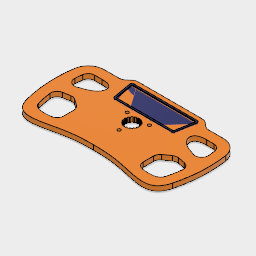
FSAE Steering Wheel 4_CSA011020 (Autodesk Fusion 360 design; units mm, degrees)
Autodesk Fusion 360 part; units mm, degrees
note: some values were not read from the file. Set by a fixed rule: which sketch regions a step uses.
sketch "Main Plate" plane through (0, 0, 0) normal (0, 1, 0) x (1, 0, 0) in component "Steering Wheel Base Plate"
  line L0 (-152.4, 0) -> (152.4, 0) construction
  line L1 (0, -76.2) -> (0, 76.2) construction
  line L2 (0, 76.2) -> (63.5, 76.2)
  line L3 (0, -76.2) -> (-8.4964, -76.2) construction
  arc A0 (144.3344, -63.5) -> (144.3344, 63.5) centre (-101.6, 0) ccw
  line L4 (88.9, 63.5) -> (144.3344, 63.5)
  spline S0 degree 5 poles (63.5, 76.2) (64.7871, 76.2) (67.2229, 75.9407) (70.4619, 74.7744) (74.1142, 71.971) (78.2858, 67.729) (81.9381, 64.9256) (85.1771, 63.7593) (87.6129, 63.5) (88.9, 63.5) knots 0 0 0 0 0 0 0.2 0.4 0.6 0.8 1 1 1 1 1 1
  spline S1 degree 5 poles (0, -76.2) (4.2797, -76.2) (12.5023, -76.2824) (23.8251, -76.6531) (37.1715, -77.6792) (52.2799, -79.9533) (67.2956, -83.1876) (83.1544, -86.9749) (99.9496, -90.4235) (115.5574, -91.6209) (128.6696, -88.7753) (136.6498, -82.0535) (141.0961, -74.0037) (143.3701, -67.235) (144.3344, -63.5) knots 0 0 0 0 0 0 0.1 0.2 0.3 0.4 0.5 0.6 0.7 0.8 0.9 1 1 1 1 1 1
  line L5 (139.5719, -81.9451) -> (149.097, -45.0549)
  line L6 (103.5148, 10.8591) -> (133.35, 0)
  arc A1 (133.35, 0) -> (129.107, 44.45) centre (-101.6, 0) ccw
  line L7 (103.707, 44.45) -> (129.107, 44.45)
  spline S2 degree 5 poles (103.707, 44.45) (99.6383, 44.45) (92.5553, 43.9266) (85.0911, 41.5729) (80.6953, 35.8381) (82.1279, 26.5542) (87.7958, 19.214) (94.5954, 14.5846) (100.3396, 12.0148) (103.5148, 10.8591) knots 0 0 0 0 0 0 0.2 0.4 0.6 0.8 1 1 1 1 1 1
  line L8 (113.232, 44.45) -> (94.182, 44.45)
  line L9 (-19.05, -76.2) -> (19.05, -76.2)
  line L10 (77.9006, -86.1433) -> (109.1683, -91.6567)
  line L11 (78.9249, -29.21) -> (78.9249, -67.31)
  arc A2 (125.8894, -58.7375) -> (132.5764, -19.05) centre (-101.6, 0) ccw
  line L12 (132.5764, -19.05) -> (101.3088, -13.5367)
  line L13 (101.3088, -13.5367) -> (78.9249, -29.21)
  spline S3 degree 5 poles (125.8894, -58.7375) (125.4726, -60.3516) (124.3156, -63.2508) (121.6104, -66.613) (116.2467, -69.3606) (106.9918, -70.6255) (97.452, -70.2137) (88.8277, -69.0979) (82.3477, -67.97) (78.9249, -67.31) knots 0 0 0 0 0 0 0.2 0.4 0.6 0.8 1 1 1 1 1 1
  line L14 (86.5574, -68.7817) -> (71.2925, -65.8383)
  line L15 (126.6342, -55.8526) -> (125.1445, -61.6224)
  line L16 (0, 76.2) -> (-63.5, 76.2)
  spline S4 degree 5 poles (-63.5, 76.2) (-64.7871, 76.2) (-67.2229, 75.9407) (-70.4619, 74.7744) (-74.1142, 71.971) (-78.2858, 67.729) (-81.9381, 64.9256) (-85.1771, 63.7593) (-87.6129, 63.5) (-88.9, 63.5) knots 0 0 0 0 0 0 0.2 0.4 0.6 0.8 1 1 1 1 1 1
  line L17 (-88.9, 63.5) -> (-144.3344, 63.5)
  spline S5 degree 5 poles (-103.707, 44.45) (-99.6383, 44.45) (-92.5553, 43.9266) (-85.0911, 41.5729) (-80.6953, 35.8381) (-82.1279, 26.5542) (-87.7958, 19.214) (-94.5954, 14.5846) (-100.3396, 12.0148) (-103.5148, 10.8591) knots 0 0 0 0 0 0 0.2 0.4 0.6 0.8 1 1 1 1 1 1
  line L18 (-113.232, 44.45) -> (-94.182, 44.45)
  line L19 (-103.707, 44.45) -> (-129.107, 44.45)
  arc A3 (-129.107, 44.45) -> (-133.35, 0) centre (101.6, 0) ccw
  line L20 (-103.5148, 10.8591) -> (-133.35, 0)
  arc A4 (-144.3344, 63.5) -> (-144.3344, -63.5) centre (101.6, 0) ccw
  spline S6 degree 5 poles (0, -76.2) (-4.2797, -76.2) (-12.5023, -76.2824) (-23.8251, -76.6531) (-37.1715, -77.6792) (-52.2799, -79.9533) (-67.2956, -83.1876) (-83.1544, -86.9749) (-99.9496, -90.4235) (-115.5574, -91.6209) (-128.6696, -88.7753) (-136.6498, -82.0535) (-141.0961, -74.0037) (-143.3701, -67.235) (-144.3344, -63.5) knots 0 0 0 0 0 0 0.1 0.2 0.3 0.4 0.5 0.6 0.7 0.8 0.9 1 1 1 1 1 1
  line L21 (19.05, -76.2) -> (-19.05, -76.2)
  line L22 (-77.9006, -86.1433) -> (-109.1683, -91.6567)
  line L23 (-139.5719, -81.9451) -> (-149.097, -45.0549)
  arc A5 (-132.5764, -19.05) -> (-125.8894, -58.7375) centre (101.6, 0) ccw
  line L24 (-132.5764, -19.05) -> (-101.3088, -13.5367)
  line L25 (-101.3088, -13.5367) -> (-78.9249, -29.21)
  line L26 (-78.9249, -29.21) -> (-78.9249, -67.31)
  spline S7 degree 5 poles (-125.8894, -58.7375) (-125.4726, -60.3516) (-124.3156, -63.2508) (-121.6104, -66.613) (-116.2467, -69.3606) (-106.9918, -70.6255) (-97.452, -70.2137) (-88.8277, -69.0979) (-82.3477, -67.97) (-78.9249, -67.31) knots 0 0 0 0 0 0 0.2 0.4 0.6 0.8 1 1 1 1 1 1
  line L27 (-126.6342, -55.8526) -> (-125.1445, -61.6224)
  line L28 (-86.5574, -68.7817) -> (-71.2925, -65.8383)
  point P0 (93.5344, -88.9)
  point P1 (-93.5344, -88.9)
  dimension "d1" = 304.8
  dimension "d2" = 152.4
  dimension "d4" = 63.5
  dimension "d5" = 254
  dimension "d6" = 12.7
  dimension "d7" = 25.4
  dimension "d8" = 38.1
  dimension "d9" = 50.8
  dimension "d10" = 25.4
  dimension "d12" = 20
  dimension "d13" = 19.05
  dimension "d14" = 19.05
  dimension "d15" = 25.4
  dimension "d16" = 31.75
  dimension "d17" = 19.05
  dimension "d18" = 38.1
  dimension "d19" = 170
  dimension "d20" = 31.75
  dimension "d22" = 19.05
  dimension "d23" = 21.59
  dimension "d24" = 10
  dimension "d25" = 19.05
  dimension "d26" = 31.75
  dimension "d27" = 135
  dimension "d28" = 38.1
  measures "d1" distance of L0.start L0.end
  measures "d2" distance of L1.start L1.end
  measures "d4" distance of L1.end L2.end
  measures "d5" radius of A0
  measures "d6" distance of L2 L4
  measures "d7" distance of L2.end L4.start
  measures "d8" distance of L5.start L5.end
  measures "d9" distance of A0.start P0
  measures "d10" distance of A0.start P0
  measures "d12" angle of L0 L6
  measures "d13" distance of A0 A1
  measures "d14" distance of L4 L7
  measures "d15" distance of A1.end L7.start
  measures "d16" distance of L6.start L6.end
  measures "d17" distance of L8.start L8.end
  measures "d18" distance of L9.start L9.end
  measures "d19" angle of L3 L10
  measures "d20" distance of L10.start L10.end
  measures "d22" distance of A0 A2
  measures "d23" distance of P0 L11.end
  measures "d24" angle of L6 L12
  measures "d25" distance of L6.end A2.end
  measures "d26" distance of A2.end L12.end
  measures "d27" angle of L12 L13
  measures "d28" distance of L11.start L11.end
sketch "Shaft Pattern" plane through (0, 0, 0) normal (0, 1, 0) x (1, 0, 0) in component "Steering Wheel Base Plate"
  circle A0 centre (0, 0) radius 12.7
  circle A1 centre (0, -25.4) radius 3.175
  circle A2 centre (21.997, 12.7) radius 3.175
  circle A3 centre (-21.997, 12.7) radius 3.175
  dimension "d34" = 25.4
  dimension "d35" = 6.35
  dimension "d36" = 25.4
  dimension "d38" = 360
  measures "d34" diameter of A0
  measures "d35" diameter of A1
  measures "d36" distance of A0.centre A1.centre
sketch "Spline" plane through (0, 0, 0) normal (0, 1, 0) x (1, 0, 0) in component "Steering Wheel Base Plate"
  line L0 (1.5875, 14.2875) -> (-1.5875, 14.2875)
  line L1 (-1.5875, 14.2875) -> (-1.5875, 11.1125)
  line L2 (-1.5875, 11.1125) -> (1.5875, 11.1125)
  line L3 (1.5875, 11.1125) -> (1.5875, 14.2875)
  line L4 (1.5875, 14.2875) -> (-1.5875, 11.1125) construction
  line L5 (-1.5875, 14.2875) -> (1.5875, 11.1125) construction
  line L6 (0, -76.2) -> (0, 76.2)
  circle A0 centre (0, 0) radius 12.7
  point P0 (0, 12.7)
  dimension "d45" = 3.175
  dimension "d46" = 3.175
  measures "d45" distance of L0.end L1.end
  measures "d46" distance of L0.start L0.end
extrude "Extrude5" add sketch "Main Plate" along normal blind 9.525 makes body 1 in component "Steering Wheel Base Plate"
extrude "Extrude6" cut sketch "Shaft Pattern" sketch "Spline" along normal through all of sketch 2 contours L2 L3 L6 A0 picked at (0.6025, -4.7194) bodies 1 in component "Steering Wheel Base Plate"
fillet "Fillet5" radius 12.7 12 edges at (-129.107, 4.7625, -44.45) (-133.35, 4.7625, 0) (-132.5764, 4.7625, 19.05) (-101.3088, 4.7625, 13.5367) (-78.9249, 4.7625, 29.21) (-78.9249, 4.7625, 67.31) (129.107, 4.7625, -44.45) (133.35, 4.7625, 0) (132.5764, 4.7625, 19.05) (101.3088, 4.7625, 13.5367) (78.9249, 4.7625, 29.21) (78.9249, 4.7625, 67.31) on bodies 1 in component "Steering Wheel Base Plate"
fillet "Fillet6" radius 31.75 2 edges at (144.3344, 4.7625, -63.5) (-144.3344, 4.7625, -63.5) on bodies 1 in component "Steering Wheel Base Plate"
extrude "Extrude7" cut sketch "Spline" along normal through all contours L0 L3 L6 A0 | L0 L1 L6 A0 | L2 L3 L6 A0 | L1 L2 L6 A0 picked at (0.8825, 11.6269) picked at (-0.606, -4.7189) bodies 1 in component "Steering Wheel Base Plate"
pattern_circular "C-Pattern1" count 16 over 360 about axis through (0, 1.75, 0) along (0, 1, 0) of "Extrude7" in component "Steering Wheel Base Plate"
sketch "Sketch4" plane through (0, 9.525, 0) normal (0, 1, 0) x (-1, 0, 0) in component "Steering Wheel Base Plate"
  line L0 (-6.9342, -12.5924) -> (-6.2886, -11.0337)
  arc A0 (-7.7873, -10.0324) -> (-6.2886, -11.0337) centre (0, 0) ccw
  line L1 (-7.7873, -10.0324) -> (-8.9803, -11.2253)
  line L2 (-8.9803, -11.2253) -> (-11.2253, -8.9803)
  line L3 (-11.2253, -8.9803) -> (-10.0324, -7.7873)
  arc A1 (-11.0337, -6.2886) -> (-10.0324, -7.7873) centre (0, 0) ccw
  line L4 (-11.0337, -6.2886) -> (-12.5924, -6.9342)
  line L5 (-12.5924, -6.9342) -> (-13.8074, -4.0009)
  line L6 (-13.8074, -4.0009) -> (-12.2488, -3.3553)
  arc A2 (-12.6004, -1.5875) -> (-12.2488, -3.3553) centre (0, 0) ccw
  line L7 (-12.6004, -1.5875) -> (-14.2875, -1.5875)
  line L8 (-14.2875, -1.5875) -> (-14.2875, 1.5875)
  line L9 (-14.2875, 1.5875) -> (-12.6004, 1.5875)
  arc A3 (-12.2488, 3.3553) -> (-12.6004, 1.5875) centre (0, 0) ccw
  line L10 (-12.2488, 3.3553) -> (-13.8074, 4.0009)
  line L11 (-13.8074, 4.0009) -> (-12.5924, 6.9342)
  line L12 (-12.5924, 6.9342) -> (-11.0337, 6.2886)
  arc A4 (-10.0324, 7.7873) -> (-11.0337, 6.2886) centre (0, 0) ccw
  line L13 (-10.0324, 7.7873) -> (-11.2253, 8.9803)
  line L14 (-11.2253, 8.9803) -> (-8.9803, 11.2253)
  line L15 (-8.9803, 11.2253) -> (-7.7873, 10.0324)
  arc A5 (-6.2886, 11.0337) -> (-7.7873, 10.0324) centre (0, 0) ccw
  line L16 (-6.2886, 11.0337) -> (-6.9342, 12.5924)
  line L17 (-6.9342, 12.5924) -> (-4.0009, 13.8074)
  line L18 (-4.0009, 13.8074) -> (-3.3553, 12.2488)
  arc A6 (-1.5875, 12.6004) -> (-3.3553, 12.2488) centre (0, 0) ccw
  line L19 (-1.5875, 12.6004) -> (-1.5875, 14.2875)
  line L20 (-1.5875, 14.2875) -> (1.5875, 14.2875)
  line L21 (1.5875, 14.2875) -> (1.5875, 12.6004)
  arc A7 (3.3553, 12.2488) -> (1.5875, 12.6004) centre (0, 0) ccw
  line L22 (3.3553, 12.2488) -> (4.0009, 13.8074)
  line L23 (4.0009, 13.8074) -> (6.9342, 12.5924)
  line L24 (6.9342, 12.5924) -> (6.2886, 11.0337)
  arc A8 (7.7873, 10.0324) -> (6.2886, 11.0337) centre (0, 0) ccw
  line L25 (7.7873, 10.0324) -> (8.9803, 11.2253)
  line L26 (8.9803, 11.2253) -> (11.2253, 8.9803)
  line L27 (11.2253, 8.9803) -> (10.0324, 7.7873)
  arc A9 (11.0337, 6.2886) -> (10.0324, 7.7873) centre (0, 0) ccw
  line L28 (11.0337, 6.2886) -> (12.5924, 6.9342)
  line L29 (12.5924, 6.9342) -> (13.8074, 4.0009)
  line L30 (13.8074, 4.0009) -> (12.2488, 3.3553)
  arc A10 (12.6004, 1.5875) -> (12.2488, 3.3553) centre (0, 0) ccw
  line L31 (12.6004, 1.5875) -> (14.2875, 1.5875)
  line L32 (14.2875, 1.5875) -> (14.2875, -1.5875)
  line L33 (14.2875, -1.5875) -> (12.6004, -1.5875)
  arc A11 (12.2488, -3.3553) -> (12.6004, -1.5875) centre (0, 0) ccw
  line L34 (12.2488, -3.3553) -> (13.8074, -4.0009)
  line L35 (13.8074, -4.0009) -> (12.5924, -6.9342)
  line L36 (12.5924, -6.9342) -> (11.0337, -6.2886)
  arc A12 (10.0324, -7.7873) -> (11.0337, -6.2886) centre (0, 0) ccw
  line L37 (10.0324, -7.7873) -> (11.2253, -8.9803)
  line L38 (11.2253, -8.9803) -> (8.9803, -11.2253)
  line L39 (8.9803, -11.2253) -> (7.7873, -10.0324)
  arc A13 (6.2886, -11.0337) -> (7.7873, -10.0324) centre (0, 0) ccw
  line L40 (6.2886, -11.0337) -> (6.9342, -12.5924)
  line L41 (6.9342, -12.5924) -> (4.0009, -13.8074)
  line L42 (4.0009, -13.8074) -> (3.3553, -12.2488)
  arc A14 (1.5875, -12.6004) -> (3.3553, -12.2488) centre (0, 0) ccw
  line L43 (1.5875, -12.6004) -> (1.5875, -14.2875)
  line L44 (1.5875, -14.2875) -> (-1.5875, -14.2875)
  line L45 (-1.5875, -14.2875) -> (-1.5875, -12.6004)
  arc A15 (-3.3553, -12.2488) -> (-1.5875, -12.6004) centre (0, 0) ccw
  line L46 (-3.3553, -12.2488) -> (-4.0009, -13.8074)
  line L47 (-4.0009, -13.8074) -> (-6.9342, -12.5924)
  arc A16 (118.3705, -63.5) -> (149.7948, -36.2857) centre (118.3705, -31.75) ccw
  arc A17 (149.7948, -36.2857) -> (144.3344, 63.5) centre (-101.6, 0) ccw
  spline S0 degree 5 poles (144.3344, 63.5) (143.3701, 67.235) (141.0961, 74.0037) (136.6498, 82.0535) (128.6696, 88.7753) (115.5574, 91.6209) (99.9496, 90.4235) (83.1544, 86.9749) (67.2956, 83.1876) (52.2799, 79.9533) (37.1715, 77.6792) (23.8251, 76.6531) (12.5023, 76.2824) (4.2797, 76.2) (0, 76.2) knots -1 -1 -1 -1 -1 -1 -0.9 -0.8 -0.7 -0.6 -0.5 -0.4 -0.3 -0.2 -0.1 0 0 0 0 0 0
  spline S1 degree 5 poles (0, 76.2) (-4.2797, 76.2) (-12.5023, 76.2824) (-23.8251, 76.6531) (-37.1715, 77.6792) (-52.2799, 79.9533) (-67.2956, 83.1876) (-83.1544, 86.9749) (-99.9496, 90.4235) (-115.5574, 91.6209) (-128.6696, 88.7753) (-136.6498, 82.0535) (-141.0961, 74.0037) (-143.3701, 67.235) (-144.3344, 63.5) knots 0 0 0 0 0 0 0.1 0.2 0.3 0.4 0.5 0.6 0.7 0.8 0.9 1 1 1 1 1 1
  arc A18 (-144.3344, 63.5) -> (-149.7948, -36.2857) centre (101.6, 0) ccw
  arc A19 (-149.7948, -36.2857) -> (-118.3705, -63.5) centre (-118.3705, -31.75) ccw
  line L48 (-118.3705, -63.5) -> (-88.9, -63.5)
  spline S2 degree 5 poles (-88.9, -63.5) (-87.6129, -63.5) (-85.1771, -63.7593) (-81.9381, -64.9256) (-78.2858, -67.729) (-74.1142, -71.971) (-70.4619, -74.7744) (-67.2229, -75.9407) (-64.7871, -76.2) (-63.5, -76.2) knots -1 -1 -1 -1 -1 -1 -0.8 -0.6 -0.4 -0.2 0 0 0 0 0 0
  line L49 (-63.5, -76.2) -> (63.5, -76.2)
  spline S3 degree 5 poles (63.5, -76.2) (64.7871, -76.2) (67.2229, -75.9407) (70.4619, -74.7744) (74.1142, -71.971) (78.2858, -67.729) (81.9381, -64.9256) (85.1771, -63.7593) (87.6129, -63.5) (88.9, -63.5) knots 0 0 0 0 0 0 0.2 0.4 0.6 0.8 1 1 1 1 1 1
  line L50 (88.9, -63.5) -> (118.3705, -63.5)
  circle A20 centre (-21.997, -12.7) radius 3.175
  circle A21 centre (21.997, -12.7) radius 3.175
  circle A22 centre (0, 25.4) radius 3.175
  arc A23 (131.2716, 31.1818) -> (125.8894, 58.7375) centre (-101.6, 0) ccw
  arc A24 (120.8893, 16.9892) -> (131.2716, 31.1818) centre (118.684, 29.4963) ccw
  line L51 (120.8893, 16.9892) -> (106.4894, 14.4501)
  arc A25 (96.9996, 16.554) -> (106.4894, 14.4501) centre (104.284, 26.9572) ccw
  line L52 (96.9996, 16.554) -> (84.3405, 25.418)
  arc A26 (78.9249, 35.8212) -> (84.3405, 25.418) centre (91.6249, 35.8212) ccw
  line L53 (78.9249, 35.8212) -> (78.9249, 56.554)
  spline S4 degree 3 poles (89.9183, 69.1388) (88.2796, 68.9165) (86.6999, 68.3764) (83.8366, 66.7209) (82.5803, 65.6214) (80.7184, 63.2084) (80.0543, 61.9718) (79.1545, 59.3328) (78.9249, 57.9481) (78.9249, 56.554) knots 0 0 0 0 0.496118 0.496118 0.992237 0.992237 1.410475 1.410475 1.828714 1.828714 1.828714 1.828714
  spline S5 degree 5 poles (89.9183, 69.1388) (90.8166, 69.2606) (94.5731, 69.7421) (100.6938, 70.3137) (108.2747, 70.4502) (116.2467, 69.3606) (121.6104, 66.613) (124.3156, 63.2508) (125.4726, 60.3516) (125.8894, 58.7375) knots -0.861384 -0.861384 -0.861384 -0.861384 -0.861384 -0.861384 -0.8 -0.6 -0.4 -0.2 0 0 0 0 0 0
  line L54 (118.3705, -44.45) -> (103.707, -44.45)
  spline S6 degree 5 poles (103.707, -44.45) (99.6383, -44.45) (92.5553, -43.9266) (85.0911, -41.5729) (80.6953, -35.8381) (82.1279, -26.5542) (87.7958, -19.214) (94.5954, -14.5846) (100.3396, -12.0148) (103.5148, -10.8591) knots 0 0 0 0 0 0 0.2 0.4 0.6 0.8 1 1 1 1 1 1
  line L55 (103.5148, -10.8591) -> (115.5421, -6.4816)
  arc A27 (132.5421, -19.468) -> (115.5421, -6.4816) centre (119.8857, -18.4157) ccw
  arc A28 (130.9402, -33.5643) -> (132.5421, -19.468) centre (-101.6, 0) ccw
  arc A29 (118.3705, -44.45) -> (130.9402, -33.5643) centre (118.3705, -31.75) ccw
  spline S7 degree 5 poles (-103.5148, -10.8591) (-100.3396, -12.0148) (-94.5954, -14.5846) (-87.7958, -19.214) (-82.1279, -26.5542) (-80.6953, -35.8381) (-85.0911, -41.5729) (-92.5553, -43.9266) (-99.6383, -44.45) (-103.707, -44.45) knots -1 -1 -1 -1 -1 -1 -0.8 -0.6 -0.4 -0.2 0 0 0 0 0 0
  line L56 (-103.707, -44.45) -> (-118.3705, -44.45)
  arc A30 (-130.9402, -33.5643) -> (-118.3705, -44.45) centre (-118.3705, -31.75) ccw
  arc A31 (-132.5421, -19.468) -> (-130.9402, -33.5643) centre (101.6, 0) ccw
  arc A32 (-115.5421, -6.4816) -> (-132.5421, -19.468) centre (-119.8857, -18.4157) ccw
  line L57 (-115.5421, -6.4816) -> (-103.5148, -10.8591)
  line L58 (-106.4894, 14.4501) -> (-120.8893, 16.9892)
  arc A33 (-131.2716, 31.1818) -> (-120.8893, 16.9892) centre (-118.684, 29.4963) ccw
  arc A34 (-125.8894, 58.7375) -> (-131.2716, 31.1818) centre (101.6, 0) ccw
  spline S8 degree 5 poles (-125.8894, 58.7375) (-125.4726, 60.3516) (-124.3156, 63.2508) (-121.6104, 66.613) (-116.2467, 69.3606) (-108.2747, 70.4502) (-100.6938, 70.3137) (-94.5731, 69.7421) (-90.8166, 69.2606) (-89.9183, 69.1388) knots 0 0 0 0 0 0 0.2 0.4 0.6 0.8 0.861384 0.861384 0.861384 0.861384 0.861384 0.861384
  spline S9 degree 3 poles (-78.9249, 56.554) (-78.9249, 58.2077) (-79.248, 59.8456) (-80.5036, 62.9054) (-81.4243, 64.2981) (-83.5653, 66.4674) (-84.7013, 67.2916) (-87.1955, 68.5379) (-88.5368, 68.9514) (-89.9183, 69.1388) knots 0 0 0 0 0.496118 0.496118 0.992237 0.992237 1.410475 1.410475 1.828714 1.828714 1.828714 1.828714
  line L59 (-78.9249, 56.554) -> (-78.9249, 35.8212)
  arc A35 (-84.3405, 25.418) -> (-78.9249, 35.8212) centre (-91.6249, 35.8212) ccw
  line L60 (-84.3405, 25.418) -> (-96.9996, 16.554)
  arc A36 (-106.4894, 14.4501) -> (-96.9996, 16.554) centre (-104.284, 26.9572) ccw
  line L61 (0, -63.5) -> (0, -41.3217) construction
  line L62 (63.5, -63.5) -> (56.7819, -25.4)
  line L63 (-56.7819, -25.4) -> (-63.5, -63.5)
  line L64 (-63.5, -63.5) -> (63.5, -63.5)
  line L65 (56.7819, -25.4) -> (23.9707, -25.4)
  line L66 (23.9707, -25.4) -> (-56.7819, -25.4)
  dimension "d56" = 63.5
  dimension "d57" = 63.5
  dimension "d58" = 80
  dimension "d59" = 80
  dimension "d60" = 12.7
  dimension "d62" = 38.1
  measures "d56" distance of L61 L63.end
  measures "d57" distance of L61 L62.start
  measures "d58" angle of L62 L64
  measures "d59" angle of L63 L64
  measures "d60" distance of L49 L64
  measures "d62" distance of L64 L66
extrude "Extrude8" add sketch "Sketch4" against normal blind 12.7 separate body contours L62 L63 L64 L65 L66 makes body 2 in component "Steering Wheel Base Plate"
sketch "Sketch5" plane through (0, 9.525, 0) normal (0, 1, 0) x (-1, 0, 0) in component "Steering Wheel Base Plate"
  line L0 (56.7819, -25.4) -> (-56.7819, -25.4)
  line L1 (-56.7819, -25.4) -> (-63.5, -63.5)
  line L2 (-63.5, -63.5) -> (63.5, -63.5)
  line L3 (63.5, -63.5) -> (56.7819, -25.4)
  line L4 (56.7819, -22.225) -> (-56.7819, -22.225)
  line L5 (-59.9087, -24.8487) -> (-66.6268, -62.9487)
  line L6 (-63.5, -66.675) -> (63.5, -66.675)
  line L7 (66.6268, -62.9487) -> (59.9087, -24.8487)
  arc A0 (63.5, -66.675) -> (66.6268, -62.9487) centre (63.5, -63.5) ccw
  arc A1 (59.9087, -24.8487) -> (56.7819, -22.225) centre (56.7819, -25.4) ccw
  arc A2 (-56.7819, -22.225) -> (-59.9087, -24.8487) centre (-56.7819, -25.4) ccw
  arc A3 (-66.6268, -62.9487) -> (-63.5, -66.675) centre (-63.5, -63.5) ccw
  dimension "d66" = 3.175
  dimension "d67" = 3.175
  dimension "d68" = 3.175
  dimension "d69" = 3.175
  dimension "d70" = 3.175
  measures "d66" radius of A0
  measures "d67" distance of L2 L6
  measures "d68" distance of L0 L4
  measures "d69" distance of L1 L5
  measures "d70" distance of L3 L7
extrude "Extrude9" add sketch "Sketch5" along normal mid plane 3.175 bodies 2 in component "Steering Wheel Base Plate"
fillet "Fillet7" radius 1.5875 4 edges at (63.5, 10.3188, -63.5) (56.7819, 10.3188, -25.4) (-63.5, 10.3188, -63.5) (-56.7819, 10.3187, -25.4) on bodies 2 in component "Steering Wheel Base Plate"
fillet "Fillet8" radius 6.35 4 edges at (-56.7819, 2.3812, -25.4) (-63.5, 2.3812, -63.5) (63.5, 2.3812, -63.5) (56.7819, 2.3812, -25.4) on bodies 2 in component "Steering Wheel Base Plate"
component "Steering Wheel Base Plate" placed x (1, 0, 0) y (0, 1, 0) z (0, 0, 1) at (0, 0, 0)
named bodies: "Plate", "Tachometer Circuit"
